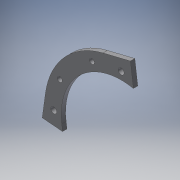
# Autodesk Inventor part: FrontMotorPlateBridge
Saved by Autodesk Inventor 2019.3 (Build 233278000, 278)
## iProperties
Created: 2019-05-08
Part Number: FrontMotorPlateBridge
Material: Generic
Document SubType Name: Modeling
Designer: eroldan
Density: 1 g/cm^3
Appearance: Default
Author: eroldan
Autodesk Inventor part; units mm, degrees
ref_plane "YZ Plane" through (0, 0, 0) normal (1, 0, 0) x (0, 1, 0)
ref_plane "XZ Plane" through (0, 0, 0) normal (0, 1, 0) x (-1, 0, 0)
ref_plane "XY Plane" through (0, 0, 0) normal (0, 0, 1) x (1, 0, 0)
sketch "Sketch1" plane through (0, 0, 0) normal (0, 0, 1) x (1, 0, 0)
  arc A0 (-18.1959, 74.3045) -> (-75.755, 10.6506) centre (0, 0) ccw
  line L0 (-78.9841, -12.3172) -> (-75.755, 10.6506)
  arc A1 (12.2439, 58.7374) -> (-59.4846, -7.8472) centre (0, 0) ccw
  line L1 (-18.1959, 74.3045) -> (9.302, 81.0383)
  line L2 (-59.4846, -7.8472) -> (-58.6652, -14.0586)
  line L3 (-78.9841, -12.3172) -> (-58.6652, -14.0586)
  line L4 (12.2439, 58.7374) -> (9.302, 81.0383)
  circle A2 centre (-67.5, 0) radius 3 projected
  circle A3 centre (0, 67.5) radius 3 projected
  circle A4 centre (52.0914, 68.8152) radius 17.05 construction
  line L5 (-32.9083, 50.1702) -> (-43.208, 63.1294) construction
  line L6 (-50.5977, 32.2471) -> (-61.3205, 45.7388) construction
  circle A5 centre (-61.4614, 29.8439) radius 2.5
  circle A6 centre (-29.2318, 61.6164) radius 2.5
  point P0 (0, 0)
  dimension "d2" = 25
  dimension "d3" = 5
  dimension "d4" = 5
  dimension "d6" = 10
  constraints: 14 end point, 8 point on circle, 4 centre point, 1 parallel, 3 other
  measures "d2" distance between parallel lines of L5 L6
  measures "d3" diameter of A5
  measures "d4" diameter of A6
  measures "d6" distance from line of A6.centre L5
extrude "Extrusion1" add sketch "Sketch1" along normal blind 4.4
body "Solid1"
